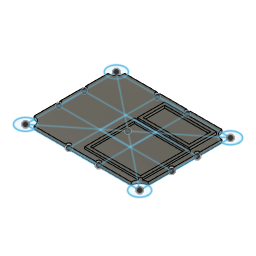
ipbox_floor (Autodesk Fusion 360 design; units mm, degrees)
Autodesk Fusion 360 part; units mm, degrees
sketch "Sketch1" plane through (0, 0, 0) normal (0, 0, 1) x (1, 0, 0)
  line L0 (-75, 75) -> (160, 75)
  line L1 (160, 75) -> (160, -112)
  line L2 (160, -112) -> (-75, -112)
  line L3 (-75, -112) -> (-75, 75)
  circle A0 centre (-75, 75) radius 17.5
  circle A1 centre (160, 75) radius 17.5
  circle A2 centre (160, -112) radius 17.5
  circle A3 centre (-75, -112) radius 17.5
  line L4 (-75, 75) -> (160, -112)
  line L5 (160, 75) -> (-75, -112)
  line L6 (73.25, -44.75) -> (11.75, -44.75)
  line L7 (11.75, -44.75) -> (11.75, 7.75)
  line L8 (11.75, 7.75) -> (73.25, 7.75)
  line L9 (73.25, 7.75) -> (73.25, -44.75)
  line L10 (73.25, -44.75) -> (11.75, 7.75) construction
  line L11 (11.75, -44.75) -> (73.25, 7.75) construction
  line L12 (11.75, 7.75) -> (11.75, -44.75)
  line L13 (11.75, -44.75) -> (-73.65, -44.75)
  line L14 (-73.65, -44.75) -> (-73.65, 7.75)
  line L15 (-73.65, 7.75) -> (11.75, 7.75)
  line L16 (73.25, 7.75) -> (73.25, -44.75)
  line L17 (73.25, -44.75) -> (158.65, -44.75)
  line L18 (158.65, -44.75) -> (158.65, 7.75)
  line L19 (158.65, 7.75) -> (73.25, 7.75)
  line L20 (11.75, 7.75) -> (73.25, 7.75)
  line L21 (73.25, 7.75) -> (73.25, 72.45)
  line L22 (73.25, 72.45) -> (11.75, 72.45)
  line L23 (11.75, 72.45) -> (11.75, 7.75)
  line L24 (11.75, -44.75) -> (73.25, -44.75)
  line L25 (73.25, -44.75) -> (73.25, -109.45)
  line L26 (73.25, -109.45) -> (11.75, -109.45)
  line L27 (11.75, -109.45) -> (11.75, -44.75)
  circle A4 centre (11.75, 72.45) radius 1.9
  circle A5 centre (73.25, 72.45) radius 1.9
  circle A6 centre (158.65, 7.75) radius 1.9
  circle A7 centre (158.65, -44.75) radius 1.9
  circle A8 centre (73.25, -109.45) radius 1.9
  circle A9 centre (11.75, -109.45) radius 1.9
  circle A10 centre (-73.65, -44.75) radius 1.9
  circle A11 centre (-73.65, 7.75) radius 1.9
  point P0 (42.5, -18.5)
  dimension "d1" = 235
  dimension "d2" = 187
  dimension "d3" = 35
  dimension "d4" = 35
  dimension "d5" = 35
  dimension "d6" = 35
  dimension "d7" = 61.5
  dimension "d8" = 52.5
  dimension "d9" = 85.4
  dimension "d10" = 85.4
  dimension "d11" = 64.7
  dimension "d12" = 64.7
  dimension "d13" = 3.8
  dimension "d14" = 3.8
  dimension "d15" = 3.8
  dimension "d16" = 3.8
  dimension "d17" = 3.8
  dimension "d18" = 3.8
  dimension "d19" = 3.8
  dimension "d20" = 3.8
  constraint horizontal L0
  constraint vertical L1
  constraint horizontal L2
  constraint vertical L3
  constraint coincident L0.start L3.end
  constraint coincident L0.end L1.start
  constraint coincident L1.end L2.start
  constraint coincident L2.end L3.start
  constraint horizontal L6
  constraint perpendicular L6 L7
  constraint parallel L6 L8
  constraint parallel L7 L9
  constraint coincident L10 P0
  constraint coincident L11 P0
  constraint midpoint L5 P0
  constraint perpendicular L12 L13
  constraint parallel L12 L14
  constraint parallel L13 L15
  constraint perpendicular L16 L17
  constraint parallel L16 L18
  constraint parallel L17 L19
  constraint perpendicular L20 L21
  constraint parallel L20 L22
  constraint parallel L21 L23
  constraint perpendicular L24 L25
  constraint parallel L24 L26
  constraint parallel L25 L27
  constraint coincident L22.end L23.start
  constraint coincident L21.end L22.start
  constraint coincident L18.end L19.start
  constraint coincident L17.end L18.start
  constraint coincident L25.end L26.start
  constraint coincident L26.end L27.start
  constraint coincident L13.end L14.start
  constraint coincident L14.end L15.start
  measures "d1" distance of L0.start L0.end
  measures "d2" distance of L0.start L2.end
  measures "d3" diameter of A0
  measures "d4" diameter of A1
  measures "d5" diameter of A2
  measures "d6" diameter of A3
  measures "d7" distance of L7.end L8.end
  measures "d8" distance of L6.end L7.end
  measures "d9" distance of L7.end L14.end
  measures "d10" distance of L8.end L18.end
  measures "d11" distance of L7.end L22.end
  measures "d12" distance of L6.end L26.end
  measures "d13" diameter of A4
  measures "d14" diameter of A5
  measures "d15" diameter of A6
  measures "d16" diameter of A7
  measures "d17" diameter of A8
  measures "d18" diameter of A9
  measures "d19" diameter of A10
  measures "d20" diameter of A11
extrude "Extrude1" add sketch "Sketch1" along normal blind 6 contours L0 A0 A1 L4 L5 L15 L19 L21 L22 L23 A4 A5 | L3 A0 L4 L15 A11 | L4 L5 L7 L12 L13 L14 L15 A10 A11 | L1 A1 L5 L19 A6 | L3 L14 A10 A11 | L4 L5 L7 L8 L9 L12 L16 L20 | L4 L5 L7 L12 | L8 L20 L21 L22 L23 A4 A5 | L4 L5 L9 L16 L17 L18 L19 A6 A7 | L4 L5 L9 L16 | L4 L5 L6 L7 L9 L12 L16 L24 | L3 A3 L5 L13 A10 | L2 A2 A3 L4 L5 L13 L17 L25 L26 L27 A8 A9 | L6 L24 L25 L26 L27 A8 A9 | L1 L18 A6 A7 | L1 A2 L4 L17 A7
chamfer "Chamfer1" distance 2.5 angle 45 8 edges at (9.9786, 73.1371, 6) (71.4786, 73.1371, 6) (-71.75, 7.75, 6) (-71.75, -44.75, 6) (156.75, 7.75, 6) (156.75, -44.75, 6) (71.4786, -108.7629, 6) (9.9786, -108.7629, 6)
extrude "Extrude2" add sketch "Sketch1" along normal blind 6 contours L4 L7 L12 L15 | L5 L9 L16 L19 | L5 L7 L12 L13 | L4 L9 L16 L17
sketch "Sketch2" plane through (0, 0, 6) normal (0, 0, 1) x (-1, 0, 0)
  arc A0 (-15.3357, 112) -> (-8.1643, 112) centre (-11.75, 109.45) ccw
  line L0 (-15.3357, 112) -> (-69.6643, 112)
  arc A1 (-76.8357, 112) -> (-69.6643, 112) centre (-73.25, 109.45) ccw
  line L1 (-76.8357, 112) -> (-142.5, 112)
  arc A2 (-160, 94.5) -> (-142.5, 112) centre (-160, 112) ccw
  line L2 (-160, 94.5) -> (-160, 48.9378)
  arc A3 (-160, 40.5622) -> (-160, 48.9378) centre (-158.65, 44.75) ccw
  line L3 (-160, 40.5622) -> (-160, -3.5622)
  arc A4 (-160, -11.9378) -> (-160, -3.5622) centre (-158.65, -7.75) ccw
  line L4 (-160, -11.9378) -> (-160, -57.5)
  arc A5 (-142.5, -75) -> (-160, -57.5) centre (-160, -75) ccw
  line L5 (-142.5, -75) -> (-76.8357, -75)
  arc A6 (-69.6643, -75) -> (-76.8357, -75) centre (-73.25, -72.45) ccw
  line L6 (-69.6643, -75) -> (-15.3357, -75)
  arc A7 (-8.1643, -75) -> (-15.3357, -75) centre (-11.75, -72.45) ccw
  line L7 (-8.1643, -75) -> (57.5, -75)
  arc A8 (75, -57.5) -> (57.5, -75) centre (75, -75) ccw
  line L8 (75, -57.5) -> (75, -11.9378)
  arc A9 (75, -3.5622) -> (75, -11.9378) centre (73.65, -7.75) ccw
  line L9 (75, -3.5622) -> (75, 40.5622)
  arc A10 (75, 48.9378) -> (75, 40.5622) centre (73.65, 44.75) ccw
  line L10 (75, 48.9378) -> (75, 94.5)
  arc A11 (57.5, 112) -> (75, 94.5) centre (75, 112) ccw
  line L11 (57.5, 112) -> (-8.1643, 112)
  line L12 (-145, 95) -> (-41.8, 95)
  line L13 (-41.8, 95) -> (-41.8, 4.4)
  line L14 (-41.8, 4.4) -> (-145, 4.4)
  line L15 (-145, 4.4) -> (-145, 95)
  line L16 (-41.8, 4.4) -> (-35.8, 4.4)
  line L17 (-35.8, 4.4) -> (-35.8, -1.6)
  line L18 (-35.8, -1.6) -> (-41.8, -1.6)
  line L19 (-41.8, -1.6) -> (-41.8, 4.4)
  line L20 (-145, 95) -> (-151, 95)
  line L21 (-151, 95) -> (-151, 101)
  line L22 (-151, 101) -> (-145, 101)
  line L23 (-145, 101) -> (-145, 95)
  line L24 (-35.8, -1.6) -> (-151, -1.6)
  line L25 (-151, -1.6) -> (-151, 101)
  line L26 (-151, 101) -> (-35.8, 101)
  line L27 (-35.8, 101) -> (-35.8, -1.6)
  dimension "d26" = 103.2
  dimension "d27" = 90.6
  dimension "d28" = 6
  dimension "d29" = 6
  dimension "d30" = 6
  dimension "d31" = 6
  constraint horizontal L12
  constraint vertical L13
  constraint horizontal L14
  constraint vertical L15
  constraint horizontal L16
  constraint vertical L17
  constraint horizontal L18
  constraint vertical L19
  constraint horizontal L20
  constraint vertical L21
  constraint horizontal L22
  constraint vertical L23
  constraint horizontal L24
  constraint vertical L25
  constraint horizontal L26
  constraint vertical L27
  measures "d26" distance of L12.start L12.end
  measures "d27" distance of L12.start L14.end
  measures "d28" distance of L13.end L16.end
  measures "d29" distance of L13.end L18.end
  measures "d30" distance of L12.start L20.end
  measures "d31" distance of L12.start L22.end
extrude "Extrude3" add sketch "Sketch2" along normal blind 4 contours A2 L20 L21 L22 L23 L25 L26 | L12 L13 L16 L23 L26 L27 | L14 L15 L19 L20 L24 L25 | L16 L17 L18 L19 L24 L27
sketch "Sketch3" plane through (0, 0, 6) normal (0, 0, 1) x (-1, 0, 0)
  line L0 (-151, -1.6) -> (-151, 96.9917)
  arc A0 (-160, 94.5) -> (-151, 96.9917) centre (-160, 112) ccw
  line L1 (-160, 94.5) -> (-160, 48.9378)
  arc A1 (-160, 40.5622) -> (-160, 48.9378) centre (-158.65, 44.75) ccw
  line L2 (-160, 40.5622) -> (-160, -3.5622)
  arc A2 (-160, -11.9378) -> (-160, -3.5622) centre (-158.65, -7.75) ccw
  line L3 (-160, -11.9378) -> (-160, -57.5)
  arc A3 (-142.5, -75) -> (-160, -57.5) centre (-160, -75) ccw
  line L4 (-142.5, -75) -> (-76.8357, -75)
  arc A4 (-69.6643, -75) -> (-76.8357, -75) centre (-73.25, -72.45) ccw
  line L5 (-69.6643, -75) -> (-15.3357, -75)
  arc A5 (-8.1643, -75) -> (-15.3357, -75) centre (-11.75, -72.45) ccw
  line L6 (-8.1643, -75) -> (57.5, -75)
  arc A6 (75, -57.5) -> (57.5, -75) centre (75, -75) ccw
  line L7 (75, -57.5) -> (75, -11.9378)
  arc A7 (75, -3.5622) -> (75, -11.9378) centre (73.65, -7.75) ccw
  line L8 (75, -3.5622) -> (75, 40.5622)
  arc A8 (75, 48.9378) -> (75, 40.5622) centre (73.65, 44.75) ccw
  line L9 (75, 48.9378) -> (75, 94.5)
  arc A9 (57.5, 112) -> (75, 94.5) centre (75, 112) ccw
  line L10 (57.5, 112) -> (-8.1643, 112)
  arc A10 (-15.3357, 112) -> (-8.1643, 112) centre (-11.75, 109.45) ccw
  line L11 (-15.3357, 112) -> (-69.6643, 112)
  arc A11 (-76.8357, 112) -> (-69.6643, 112) centre (-73.25, 109.45) ccw
  line L12 (-76.8357, 112) -> (-142.5, 112)
  arc A12 (-146.3893, 101) -> (-142.5, 112) centre (-160, 112) ccw
  line L13 (-146.3893, 101) -> (-35.8, 101)
  line L14 (-35.8, 101) -> (-35.8, -1.6)
  line L15 (-35.8, -1.6) -> (-151, -1.6)
  line L16 (-140, -10) -> (-45.3, -10)
  line L17 (-45.3, -10) -> (-45.3, -54.2)
  line L18 (-45.3, -54.2) -> (-140, -54.2)
  line L19 (-140, -54.2) -> (-140, -10)
  line L20 (-45.3, -54.2) -> (-39.3, -54.2)
  line L21 (-39.3, -54.2) -> (-39.3, -60.2)
  line L22 (-39.3, -60.2) -> (-45.3, -60.2)
  line L23 (-45.3, -60.2) -> (-45.3, -54.2)
  line L24 (-140, -10) -> (-146, -10)
  line L25 (-146, -10) -> (-146, -4)
  line L26 (-146, -4) -> (-140, -4)
  line L27 (-140, -4) -> (-140, -10)
  line L28 (-39.3, -60.2) -> (-146, -60.2)
  line L29 (-146, -60.2) -> (-146, -4)
  line L30 (-146, -4) -> (-39.3, -4)
  line L31 (-39.3, -4) -> (-39.3, -60.2)
  dimension "d34" = 94.7
  dimension "d35" = 44.2
  dimension "d36" = 6
  dimension "d37" = 6
  dimension "d38" = 6
  dimension "d39" = 6
  constraint horizontal L16
  constraint vertical L17
  constraint horizontal L18
  constraint vertical L19
  constraint horizontal L20
  constraint vertical L21
  constraint horizontal L22
  constraint vertical L23
  constraint horizontal L24
  constraint vertical L25
  constraint horizontal L26
  constraint vertical L27
  constraint horizontal L28
  constraint vertical L29
  constraint horizontal L30
  constraint vertical L31
  measures "d34" distance of L16.start L16.end
  measures "d35" distance of L16.start L18.end
  measures "d36" distance of L17.end L20.end
  measures "d37" distance of L17.end L22.end
  measures "d38" distance of L16.start L24.end
  measures "d39" distance of L16.start L26.end
extrude "Extrude4" add sketch "Sketch3" along normal blind 5 contours L16 L17 L20 L27 L30 L31 | L18 L19 L23 L24 L28 L29 | L24 L25 L26 L27 L29 L30 | L20 L21 L22 L23 L28 L31
